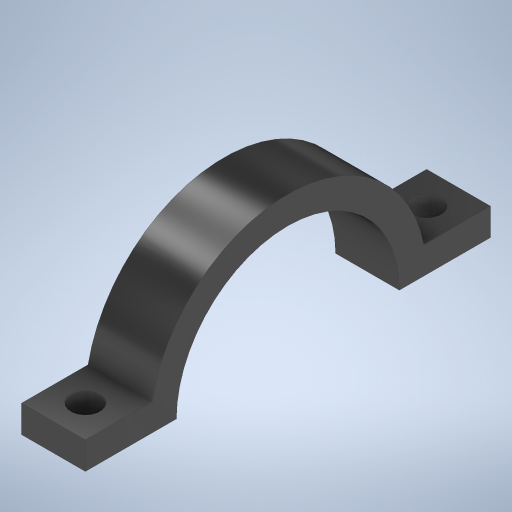
# Autodesk Inventor part: klemme
Saved by Autodesk Inventor 2023 (Build 270158000, 158)
## iProperties
Created: 2024-03-05
Part Number: klemme
Material: Generisch
Document SubType Name: Modeling
Designer: phili
Density: 1 g/cm^3
Appearance: Vorgabe
Author: phili
Autodesk Inventor part; units mm, degrees
ref_plane "YZ Plane" through (0, 0, 0) normal (1, 0, 0) x (0, 1, 0)
ref_plane "XZ Plane" through (0, 0, 0) normal (0, 1, 0) x (-1, 0, 0)
ref_plane "XY Plane" through (0, 0, 0) normal (0, 0, 1) x (1, 0, 0)
sketch "Skizze1" plane through (0, 0, 0) normal (1, 0, 0) x (0, 1, 0)
  arc A0 (0, -12.25) -> (0, 12.25) centre (0, 0) ccw
  line L0 (0, 0) -> (0, 12.25) construction
  line L1 (0, 0) -> (0, -12.25) construction
  arc A1 (0, -15.25) -> (0, 15.25) centre (0, 0) ccw
  line L2 (0, 15.25) -> (0, 12.25)
  line L3 (0, -12.25) -> (0, -15.25)
  dimension "d0" = 12.25
  dimension "d1" = 180
  dimension "d3" = 15.25
  constraints: 8 end point, 4 point on circle, 2 centre point, 2 coincident, 2 point on line, 1 vertical
  measures "d0" radius of A0
  measures "d1" angle of L1 L0
  measures "d3" radius of A1
extrude "Extrusion1" add sketch "Skizze1" along normal blind 7
sketch "Skizze3" plane through (7, 0, 0) normal (1, 0, 0) x (0, 0, -1)
  arc A0 (15.25, 0) -> (-15.25, 0) centre (0, 0) ccw projected
  line L0 (-15.25, 0) -> (-22.25, 0)
  line L1 (-22.25, 0) -> (-22.25, 3)
  line L2 (-22.25, 3) -> (-14.952, 3)
  dimension "d6" = 7
  dimension "d7" = 3
  constraints: 6 end point, 2 perpendicular, 1 horizontal, 1 point on circle
  measures "d6" distance of L0.start L0.end
  measures "d7" distance of L0.end L1.end
extrude "Extrusion3" add sketch "Skizze3" against normal blind 7
sketch "Skizze5" plane through (0, 0, 12.25) normal (0, -1, 0) x (1, 0, 0)
  line L0 (7, 10) -> (7, 0) projected
  line L1 (7, 10) -> (0, 10) projected
  point P0 (0, -12.25)
  point P1 (3.5, 6.5)
  dimension "d19" = 3.5
  dimension "d20" = 3.5
  measures "d19" distance from line of L0 point (3.5, 6.5)
  measures "d20" distance from line of point (3.5, 6.5) L1
hole "Bohrung1" at (3.5, 0, 18.75) direction (0, 1, 0) diameter 3.2 end through all
mirror "Spiegeln1" about plane through (0, 0, 0) normal (0, 0, 1) of "Extrusion3", "Bohrung1"
